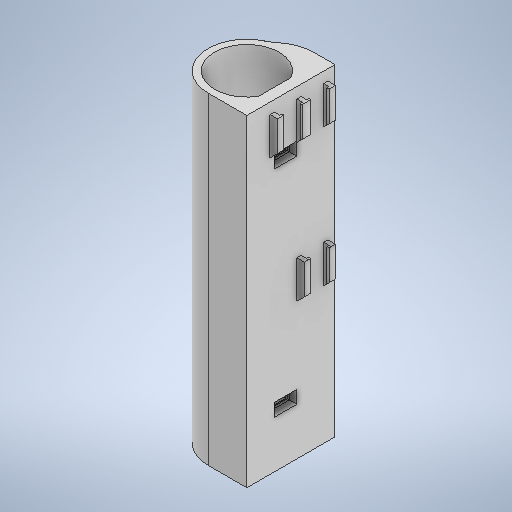
# Autodesk Inventor part: Open_source_chronograph_main_body_v2.0
Saved by Autodesk Inventor 2025 (Build 290162000, 162)
## iProperties
Created: 2025-04-15
Part Number: Open_source_chronograph_main_body_v2.0
Material: Generic
Document SubType Name: Modeling
Designer: Anarxus
Density: 1 g/cm^3
Appearance: Default
Author: Anarxus
Autodesk Inventor part; units mm, degrees
ref_plane "YZ Plane" through (0, 0, 0) normal (1, 0, 0) x (0, 1, 0)
ref_plane "XZ Plane" through (0, 0, 0) normal (0, 1, 0) x (-1, 0, 0)
ref_plane "XY Plane" through (0, 0, 0) normal (0, 0, 1) x (1, 0, 0)
sketch "Sketch1" plane through (0, 0, 0) normal (0, 1, 0) x (-1, 0, 0)
  circle A0 centre (0, 0) radius 15
  circle A1 centre (0, 0) radius 18
  line L0 (-15, 0) -> (-13, 0)
  line L1 (-13, 0) -> (-13, -7.4833)
  line L2 (-13, 0) -> (-13, 7.4833)
  line L3 (-18, 0) -> (-18, 18)
  line L4 (-18, 18) -> (0, 18)
  line L5 (-18, 0) -> (-18, -23)
  line L6 (-18, -23) -> (0, -23)
  line L7 (0, -23) -> (0, -18)
  dimension "d0" = 30
  dimension "d1" = 3
  dimension "d3" = 2
  dimension "d4" = 23
  dimension "d7" = 18
  constraints: 16 end point, 6 point on circle, 4 vertical, 3 perpendicular, 2 centre point, 2 tangent, 1 coincident, 1 horizontal
  measures "d0" diameter of A0
  measures "d1" radial gap between concentric circles of A0 A1
  measures "d3" distance of L0.start L0.end
  measures "d4" distance of L3.start L5.end
  measures "d7" distance of L3.start L3.end
extrude "Extrusion1" add sketch "Sketch1" along normal blind 150 contours L2 L0 A0 | A0 L0 L1 | A1 | A1 L3 L4 | L7 L6 L5 A1
sketch "Sketch2" plane through (18, 0, 18) normal (1, 0, 0) x (0, 0, -1)
  line L0 (0, 0) -> (18, 0)
  line L1 (18, 0) -> (18, 158.8322)
  line L2 (0, 150) -> (41, 150) projected
  line L3 (18, 150) -> (18, 125)
  line L4 (18, 0) -> (18, 25)
  line L5 (18, 125) -> (18, 122)
  line L6 (18, 122) -> (23.25, 122)
  line L7 (23.25, 122) -> (23.25, 128)
  line L8 (23.25, 128) -> (12.75, 128)
  line L9 (12.75, 128) -> (12.75, 122)
  line L10 (12.75, 122) -> (18, 122)
  line L11 (18, 125) -> (18, 123)
  line L12 (18, 123) -> (22, 123)
  line L13 (22, 123) -> (22, 127)
  line L14 (22, 127) -> (14, 127)
  line L15 (14, 127) -> (14, 123)
  line L16 (14, 123) -> (18, 123)
  line L17 (23.25, 22) -> (23.25, 28)
  line L18 (18, 22) -> (23.25, 22)
  line L19 (12.75, 22) -> (18, 22)
  line L20 (12.75, 28) -> (12.75, 22)
  line L21 (23.25, 28) -> (12.75, 28)
  line L22 (22, 27) -> (14, 27)
  line L23 (14, 23) -> (18, 23)
  line L24 (22, 23) -> (22, 27)
  line L25 (14, 27) -> (14, 23)
  line L26 (18, 23) -> (22, 23)
  dimension "d8" = 25
  dimension "d9" = 25
  dimension "d10" = 3
  dimension "d11" = 5.25
  dimension "d12" = 6
  dimension "d13" = 10.5
  dimension "d14" = 2
  dimension "d15" = 4
  dimension "d16" = 4
  dimension "d17" = 8
  dimension "d20" = 100
  constraints: 52 end point, 10 perpendicular, 8 point on line, 2 horizontal, 1 vertical, 20 other
  measures "d8" distance of L3.start L3.end
  measures "d9" distance of L0.end L4.end
  measures "d10" distance of L3.end L5.end
  measures "d11" distance of L5.end L6.end
  measures "d12" distance of L6.end L7.end
  measures "d13" distance of L7.end L8.end
  measures "d14" distance of L3.end L11.end
  measures "d15" distance of L11.end L12.end
  measures "d16" distance of L12.end L13.end
  measures "d17" distance of L13.end L14.end
  measures "d20" distance of L6.end L17.start
extrude "Extrusion2" cut sketch "Sketch2" against normal blind 10.5 contours L23 L25 L22 L1 | L1 L22 L24 L26 | L16 L15 L14 L1 | L1 L14 L13 L12
extrude "Extrusion3" cut sketch "Sketch2" against normal blind 4 contours L19 L20 L21 L1 L22 L25 L23 | L1 L26 L24 L22 L21 L17 L18 | L10 L9 L8 L1 L14 L15 L16 | L1 L12 L13 L14 L8 L7 L6
fillet "Fillet1" radius 0.5 8 edges at (14, 125, -5.25) (14, 122, 0) (14, 128, 0) (14, 125, 5.25) (14, 25, 5.25) (14, 22, 0) (14, 28, 0) (14, 25, -5.25)
sketch "Sketch3" plane through (18, 0, 18) normal (1, 0, 0) x (0, 0, -1)
  line L0 (23.25, 128) -> (23.25, 122) projected
  line L1 (23.25, 128) -> (23.25, 150.2254)
  line L2 (12.75, 122) -> (12.75, 128) projected
  line L3 (12.75, 128) -> (12.75, 150)
  line L4 (0, 150) -> (41, 150) projected
  line L5 (12.75, 128) -> (12.75, 131)
  line L6 (12.75, 131) -> (10.75, 131)
  line L7 (10.75, 131) -> (10.75, 145)
  line L8 (10.75, 145) -> (12.75, 145)
  line L9 (23.25, 131) -> (25.25, 131)
  line L10 (25.25, 131) -> (25.25, 145)
  line L11 (25.25, 145) -> (23.25, 145)
  line L12 (25.25, 145) -> (35.75, 145)
  line L13 (35.75, 145) -> (37.75, 145)
  line L14 (37.75, 145) -> (37.75, 131)
  line L15 (37.75, 131) -> (35.75, 131)
  line L16 (35.75, 131) -> (35.75, 145)
  line L17 (37.75, 131) -> (37.75, 81)
  line L18 (37.75, 81) -> (37.75, 67)
  line L19 (37.75, 67) -> (35.75, 67)
  line L20 (35.75, 67) -> (35.75, 81)
  line L21 (35.75, 81) -> (37.75, 81)
  line L22 (25.25, 81) -> (25.25, 67)
  line L23 (23.25, 67) -> (23.25, 81)
  line L24 (23.25, 81) -> (25.25, 81)
  line L25 (25.25, 67) -> (23.25, 67)
  line L26 (35.75, 145) -> (36, 45.0003)
  line L27 (36, 0) -> (36, 150) projected
  point P0 (18, 0)
  dimension "d30" = 3
  dimension "d31" = 2
  dimension "d32" = 14
  dimension "d33" = 2
  dimension "d34" = 10.5
  dimension "d35" = 2
  dimension "d36" = 50
  dimension "d37" = 14
  dimension "d54" = 100
  constraints: 48 end point, 19 point on line, 9 perpendicular, 3 parallel, 3 vertical, 1 horizontal
  measures "d30" distance of L2.end L5.end
  measures "d31" distance of L5.end L6.end
  measures "d32" distance of L6.end L7.end
  measures "d33" distance of L9.start L9.end
  measures "d34" distance of L10.end L12.end
  measures "d35" distance of L12.end L13.end
  measures "d36" distance of L14.end L17.end
  measures "d37" distance of L17.end L18.end
  measures "d54" distance of L12.end L26.end
extrude "Extrusion4" add sketch "Sketch3" along normal blind 3.5 contours L1 L11 L10 L9 | L26 L15 L16 | L13 L27 L15 L26 | L13 L14 L15 L27 | L26 L19 L20 L21 | L21 L27 L19 L26 | L21 L18 L19 L27 | L6 L7 L8 L3 | L22 L25 L23 L24
sketch "Sketch4" plane through (18, 131, -17.75) normal (0, 0, 1) x (1, 0, 0)
  line L0 (0, 14) -> (2.5, 14)
  line L1 (0, 14) -> (3.5, 14) projected
  line L2 (3.5, 14) -> (3.5, 0) projected
  line L3 (2.5, 14) -> (3.5, 14)
  line L4 (3.5, 14) -> (3.5, 0)
  line L5 (3.5, 0) -> (2.5, 0)
  line L6 (2.5, 0) -> (2.5, 14)
  line L7 (0, -64) -> (3.5, -64) projected
  line L8 (3.5, -49.9886) -> (2.5, -49.9886)
  line L9 (2.5, -49.9886) -> (2.5, -64)
  line L10 (2.5, -64) -> (3.5, -64)
  line L11 (3.5, -64) -> (3.5, -49.9886)
  point P0 (-18, -131)
  dimension "d40" = 2.5
  dimension "d41" = 1
  constraints: 18 end point, 4 parallel, 3 point on line, 2 horizontal, 2 perpendicular
  measures "d40" distance of L0.start L0.end
  measures "d41" distance of L10.end L9.end
extrude "Extrusion5" add sketch "Sketch4" along normal blind 1
sketch "Sketch5" plane through (18, 131, -7.25) normal (0, 0, -1) x (-1, 0, 0)
  line L0 (0, 14) -> (-3.5, 14) projected
  line L1 (0, 0) -> (-3.5, 0) projected
  line L2 (-3.5, 14) -> (-2.5, 14)
  line L3 (-2.5, 14) -> (-2.5, 0)
  line L4 (-2.5, 0) -> (-3.5, 0)
  line L5 (-3.5, 0) -> (-3.5, 14)
  line L6 (0, -64) -> (-3.5, -64) projected
  line L7 (-3.5, -50.0135) -> (-2.5, -50.0135)
  line L8 (-2.5, -50.0135) -> (-2.5, -64)
  line L9 (-2.5, -64) -> (-3.5, -64)
  line L10 (-3.5, -64) -> (-3.5, -50.0135)
  point P0 (18, -131)
  point P1 (-2.5, 14)
  dimension "d44" = 1
  dimension "d45" = 1
  constraints: 16 end point, 4 parallel, 3 point on line, 2 horizontal, 2 perpendicular
  measures "d44" distance of L3.end L4.end
  measures "d45" distance of L8.end L9.end
extrude "Extrusion6" add sketch "Sketch5" along normal blind 1
sketch "Sketch6" plane through (18, 131, -5.25) normal (0, 0, 1) x (1, 0, 0)
  line L0 (3.5, 14) -> (3.5, 0) projected
  line L1 (2.5, 14) -> (2.5, 0) projected
  line L2 (3.5, 14) -> (2.5, 14)
  line L3 (2.5, 14) -> (2.5, 0)
  line L4 (2.5, 0) -> (3.5, 0)
  line L5 (3.5, 0) -> (3.5, 14)
  point P0 (-18, -131)
  dimension "d48" = 1
  constraints: 8 end point, 2 parallel, 1 horizontal, 1 perpendicular
  measures "d48" distance of L4.end L1.end
extrude "Extrusion7" add sketch "Sketch6" along normal blind 1
sketch "Sketch7" plane through (18, 131, 5.25) normal (0, 0, -1) x (-1, 0, 0)
  line L0 (-3.5, 0) -> (-3.5, 14) projected
  line L1 (-3.5, 14) -> (-2.5, 14)
  line L2 (-2.5, 14) -> (-2.5, 0)
  line L3 (-2.5, 0) -> (-3.5, 0)
  line L4 (-3.5, 0) -> (-3.5, 14)
  point P0 (18, -131)
  dimension "d51" = 1
  constraints: 8 end point, 2 parallel, 1 horizontal, 1 perpendicular
  measures "d51" distance of L2.end L3.end
extrude "Extrusion8" add sketch "Sketch7" along normal blind 1
fillet "Fillet2" radius 20 2 edges at (0, 75, -18) (0, 75, -23)
chamfer "Chamfer1" distance 3.5 angle 45 5 edges at (18, 131, -6.25) (18, 131, -18.75) (18, 131, 6.25) (18, 67, -18.75) (18, 67, -6.25)
equation "\"d25\" = d13"
body "Solid1"
